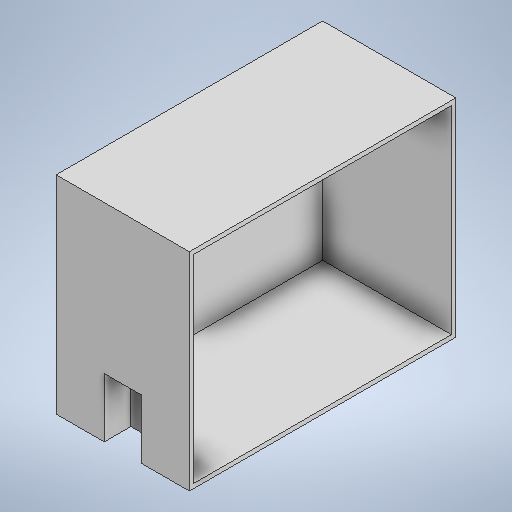
# Autodesk Inventor part: Self_balancing_robot
Saved by Autodesk Inventor 2025 (Build 290162000, 162)
## iProperties
Created: 2025-06-27
Part Number: Self_balancing_robot
Material: Generic
Document SubType Name: Modeling
Designer: joann
Density: 1 g/cm^3
Appearance: Default
Author: joann
Autodesk Inventor part; units mm, degrees
ref_plane "YZ Plane" through (0, 0, 0) normal (1, 0, 0) x (0, 1, 0)
ref_plane "XZ Plane" through (0, 0, 0) normal (0, 1, 0) x (-1, 0, 0)
ref_plane "XY Plane" through (0, 0, 0) normal (0, 0, 1) x (1, 0, 0)
sketch "Sketch1" plane through (0, 0, 0) normal (0, 1, 0) x (-1, 0, 0)
  line L0 (45, 90) -> (-45, 90)
  line L1 (-45, 90) -> (-45, -90)
  line L2 (-45, -90) -> (45, -90)
  line L3 (45, -90) -> (45, 90)
  point P0 (0, 0)
  dimension "d0" = 180
  dimension "d1" = 90
  dimension "d2" = 45
  dimension "d3" = 90
  constraints: 8 end point, 2 parallel, 1 horizontal, 1 perpendicular
  measures "d0" distance of L0.end L1.end
  measures "d1" distance of L1.end L2.end
  measures "d2" distance from line of L1 point (0, 0)
  measures "d3" distance from line of L2 point (0, 0)
extrude "Extrusion1" add sketch "Sketch1" along normal blind 140
sketch "Sketch2" plane through (45, 0, 90) normal (1, 0, 0) x (0, 0, -1)
  line L0 (3, 137) -> (177, 137)
  line L1 (177, 137) -> (177, 3)
  line L2 (177, 3) -> (3, 3)
  line L3 (3, 3) -> (3, 137)
  line L4 (0, 140) -> (180, 140) projected
  line L5 (0, 0) -> (0, 140) projected
  point P0 (90, 0)
  dimension "d6" = 3
  dimension "d7" = 3
  dimension "d8" = 174
  dimension "d9" = 134
  constraints: 8 end point, 2 parallel, 1 horizontal, 1 perpendicular
  measures "d6" distance between parallel lines of L4 L0
  measures "d7" distance between parallel lines of L5 L3
  measures "d8" distance between parallel lines of L1 L3
  measures "d9" distance between parallel lines of L2 L0
extrude "Extrusion2" cut sketch "Sketch2" against normal blind 87
sketch "Sketch3" plane through (-45, 0, 90) normal (0, 0, 1) x (1, 0, 0)
  line L0 (90, 0) -> (0, 0) projected
  line L1 (32.5, 40) -> (57.5, 40)
  line L2 (57.5, 40) -> (57.5, 0)
  line L3 (57.5, 0) -> (32.5, 0)
  line L4 (32.5, 0) -> (32.5, 40)
  line L5 (90, 0) -> (90, 140) projected
  point P0 (45, 0)
  point P1 (57.5, 20)
  point P2 (32.5, 20)
  dimension "d12" = 25
  dimension "d13" = 32.5
  dimension "d14" = 40
  constraints: 8 end point, 2 midpoint, 2 parallel, 1 horizontal, 1 perpendicular, 1 point on line
  measures "d12" distance of point (57.5, 20) point (32.5, 20)
  measures "d13" distance between parallel lines of L5 L2
  measures "d14" distance between parallel lines of L0 L1
sketch "Sketch4" plane through (-45, 0, 90) normal (0, 0, 1) x (1, 0, 0)
  line L0 (90, 0) -> (0, 0) projected
  line L1 (30.5, 41.9359) -> (59.5, 41.9359)
  line L2 (59.5, 41.9359) -> (59.5, 0)
  line L3 (59.5, 0) -> (30.5, 0)
  line L4 (30.5, 0) -> (30.5, 41.9359)
  line L5 (90, 0) -> (90, 140) projected
  point P0 (45, 0)
  dimension "d15" = 29
  dimension "d16" = 30.5
  constraints: 8 end point, 2 parallel, 1 horizontal, 1 perpendicular, 1 point on line
  measures "d15" distance between parallel lines of L2 L4
  measures "d16" distance between parallel lines of L5 L2
extrude "Extrusion3" add sketch "Sketch4" against normal blind 20
extrude "Extrusion4" cut sketch "Sketch3" against normal blind 18
body "Solid1"
